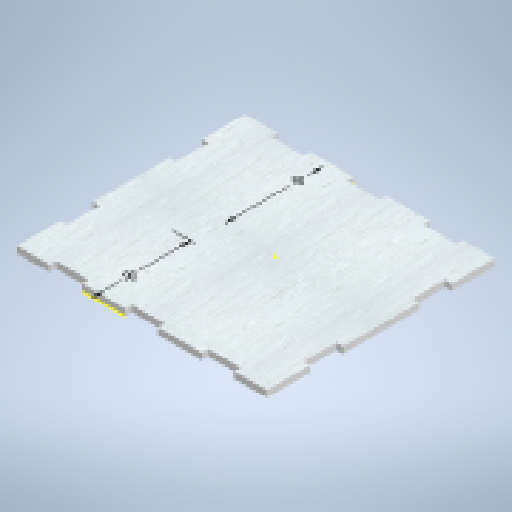
# Autodesk Inventor part: Низ робота
Saved by Autodesk Inventor 2024.2 (Build 282272000, 272)
## iProperties
Created: 2026-01-27
Part Number: Низ робота
Material: Типовые
Document SubType Name: Modeling
Designer: Service
Density: 1 g/cm^3
Appearance: По умолчанию
Author: Service
Autodesk Inventor part; units mm, degrees
ref_plane "YZ Plane" through (0, 0, 0) normal (1, 0, 0) x (0, 1, 0)
ref_plane "XZ Plane" through (0, 0, 0) normal (0, 1, 0) x (-1, 0, 0)
ref_plane "XY Plane" through (0, 0, 0) normal (0, 0, 1) x (1, 0, 0)
sketch "Эскиз1" plane through (0, 0, 0) normal (0, 1, 0) x (-1, 0, 0)
  line L0 (127.5386, 109.5005) -> (-102.4614, 109.5005)
  line L1 (-102.4614, 109.5005) -> (-102.4614, -100.4995)
  line L2 (-102.4614, -100.4995) -> (127.5386, -100.4995)
  line L3 (127.5386, -100.4995) -> (127.5386, 109.5005)
  line L4 (127.5386, -100.4995) -> (97.5386, -100.4995)
  line L5 (97.5386, -100.4995) -> (97.5386, -94.4995)
  line L6 (97.5386, -94.4995) -> (127.5386, -94.4995)
  line L7 (127.5386, -94.4995) -> (127.5386, -100.4995)
  line L8 (97.5386, -94.4995) -> (67.5386, -94.4995)
  line L9 (67.5386, -94.4995) -> (67.5386, -100.4995)
  line L10 (67.5386, -100.4995) -> (97.5386, -100.4995)
  line L11 (97.5386, -100.4995) -> (97.5386, -94.4995)
  line L12 (6.9803, -100.4995) -> (67.5386, -100.4995)
  line L13 (67.5386, -100.4995) -> (67.5386, -94.4995)
  line L14 (-42.4614, -94.4995) -> (-42.4614, -100.4995)
  line L15 (-42.4614, -100.4995) -> (-2.4614, -100.4995)
  line L16 (-42.4614, -94.4995) -> (-72.4614, -94.4995)
  line L17 (-72.4614, -94.4995) -> (-72.4614, -100.4995)
  line L18 (-72.4614, -100.4995) -> (-42.4614, -100.4995)
  line L19 (-42.4614, -100.4995) -> (-42.4614, -94.4995)
  line L20 (-72.4614, -94.4995) -> (-102.4614, -94.4995)
  line L21 (-102.4614, -94.4995) -> (-102.4614, -100.4995)
  line L22 (-102.4614, -100.4995) -> (-72.4614, -100.4995)
  line L23 (-72.4614, -100.4995) -> (-72.4614, -94.4995)
  line L24 (-42.4614, -94.4995) -> (-2.4614, -94.4995)
  line L25 (-2.4614, -94.4995) -> (-2.4614, -100.4995)
  line L26 (-2.4614, -100.4995) -> (-42.4614, -100.4995)
  line L27 (-42.4614, -100.4995) -> (-42.4614, -94.4995)
  line L28 (-2.4614, -100.4995) -> (27.5386, -100.4995)
  line L29 (27.5386, -100.4995) -> (27.5386, -94.4995)
  line L30 (27.5386, -94.4995) -> (-2.4614, -94.4995)
  line L31 (-2.4614, -94.4995) -> (-2.4614, -100.4995)
  line L32 (67.5386, -94.4995) -> (27.5386, -94.4995)
  line L33 (27.5386, -94.4995) -> (27.5386, -100.4995)
  line L34 (27.5386, -100.4995) -> (67.5386, -100.4995)
  line L35 (67.5386, -100.4995) -> (67.5386, -94.4995)
  line L36 (-102.4614, 103.5005) -> (127.5386, 103.5005)
  line L37 (127.5386, 103.5005) -> (97.5386, 103.5005)
  line L38 (97.5386, 103.5005) -> (97.5386, 109.5005)
  line L39 (97.5386, 109.5005) -> (127.5386, 109.5005)
  line L40 (127.5386, 109.5005) -> (127.5386, 103.5005)
  line L41 (97.5386, 109.5005) -> (67.5386, 109.5005)
  line L42 (67.5386, 109.5005) -> (67.5386, 103.5005)
  line L43 (67.5386, 103.5005) -> (97.5386, 103.5005)
  line L44 (97.5386, 103.5005) -> (97.5386, 109.5005)
  line L45 (6.9803, 103.5005) -> (67.5386, 103.5005)
  line L46 (67.5386, 103.5005) -> (67.5386, 109.5005)
  line L47 (-42.4614, 109.5005) -> (-42.4614, 103.5005)
  line L48 (-42.4614, 103.5005) -> (-2.4614, 103.5005)
  line L49 (-42.4614, 109.5005) -> (-72.4614, 109.5005)
  line L50 (-72.4614, 109.5005) -> (-72.4614, 103.5005)
  line L51 (-72.4614, 103.5005) -> (-42.4614, 103.5005)
  line L52 (-42.4614, 103.5005) -> (-42.4614, 109.5005)
  line L53 (-72.4614, 109.5005) -> (-102.4614, 109.5005)
  line L54 (-102.4614, 109.5005) -> (-102.4614, 103.5005)
  line L55 (-102.4614, 103.5005) -> (-72.4614, 103.5005)
  line L56 (-72.4614, 103.5005) -> (-72.4614, 109.5005)
  line L57 (-42.4614, 109.5005) -> (-2.4614, 109.5005)
  line L58 (-2.4614, 109.5005) -> (-2.4614, 103.5005)
  line L59 (-2.4614, 103.5005) -> (-42.4614, 103.5005)
  line L60 (-42.4614, 103.5005) -> (-42.4614, 109.5005)
  line L61 (-2.4614, 103.5005) -> (27.5386, 103.5005)
  line L62 (27.5386, 103.5005) -> (27.5386, 109.5005)
  line L63 (27.5386, 109.5005) -> (-2.4614, 109.5005)
  line L64 (-2.4614, 109.5005) -> (-2.4614, 103.5005)
  line L65 (67.5386, 109.5005) -> (27.5386, 109.5005)
  line L66 (27.5386, 109.5005) -> (27.5386, 103.5005)
  line L67 (27.5386, 103.5005) -> (67.5386, 103.5005)
  line L68 (67.5386, 103.5005) -> (67.5386, 109.5005)
  line L69 (-102.4614, 69.5005) -> (-96.4614, 69.5005)
  line L70 (-96.4614, 69.5005) -> (-96.4614, 39.5005)
  line L71 (-96.4614, 39.5005) -> (-102.4614, 39.5005)
  line L72 (-102.4614, 39.5005) -> (-102.4614, 69.5005)
  line L73 (-102.4614, -30.4995) -> (-96.4614, -30.4995)
  line L74 (-96.4614, -30.4995) -> (-96.4614, -60.4995)
  line L75 (-96.4614, -60.4995) -> (-102.4614, -60.4995)
  line L76 (-102.4614, -60.4995) -> (-102.4614, -30.4995)
  line L77 (127.5386, 69.5005) -> (121.5386, 69.5005)
  line L78 (121.5386, 69.5005) -> (121.5386, 39.5005)
  line L79 (121.5386, 39.5005) -> (127.5386, 39.5005)
  line L80 (127.5386, 39.5005) -> (127.5386, 69.5005)
  line L81 (127.5386, -30.4995) -> (121.5386, -30.4995)
  line L82 (121.5386, -30.4995) -> (121.5386, -60.4995)
  line L83 (121.5386, -60.4995) -> (127.5386, -60.4995)
  line L84 (127.5386, -60.4995) -> (127.5386, -30.4995)
  point P0 (0, 0)
  point P1 (-42.4614, -97.4995)
  point P2 (67.5386, -97.4995)
  point P3 (-42.4614, 106.5005)
  point P4 (67.5386, 106.5005)
  point P5 (-99.4614, -60.4995)
  point P6 (-2.4614, -100.4995)
  point P7 (124.5386, 69.5005)
  point P8 (124.5386, -60.4995)
  dimension "d0" = 230
  dimension "d1" = 210
  dimension "d2" = 6
  dimension "d3" = 30
  dimension "d4" = 30
  dimension "d5" = 30
  dimension "d6" = 30
  dimension "d8" = 40
  dimension "d10" = 40
  dimension "d11" = 230
  dimension "d13" = 6
  dimension "d14" = 30
  dimension "d15" = 30
  dimension "d16" = 30
  dimension "d17" = 30
  dimension "d18" = 40
  dimension "d19" = 40
  dimension "d20" = 40
  dimension "d21" = 30
  dimension "d22" = 40
  dimension "d23" = 30
  dimension "d24" = 6
  dimension "d27" = 6
  dimension "d28" = 40
  dimension "d29" = 40
  dimension "d30" = 30
  dimension "d31" = 30
  constraints: 170 end point, 38 parallel, 19 horizontal, 19 perpendicular, 16 point on line, 7 midpoint
  measures "d0" distance of L1.end L2.end
  measures "d1" distance of L0.end L1.end
  measures "d2" distance of L4.end L5.end
  measures "d3" distance of L5.end L6.end
  measures "d4" distance of L16.end L20.end
  measures "d5" distance of L14.start L16.end
  measures "d6" distance of L5.end L8.end
  measures "d8" distance of L8.end L32.end
  measures "d10" distance of L14.start L24.end
  measures "d11" distance of L55.start L40.end
  measures "d13" distance of L38.start L41.start
  measures "d14" distance of L41.start L39.end
  measures "d15" distance of L53.start L53.end
  measures "d16" distance of L57.start L53.start
  measures "d17" distance of L41.start L42.start
  measures "d18" distance of L42.start L66.start
  measures "d19" distance of L57.start L57.end
  measures "d20" distance from line of point (-99.461, -60.5) L2
  measures "d21" distance of L73.end L74.end
  measures "d22" distance between parallel lines of L69 L0
  measures "d23" distance of L69.end L70.end
  measures "d24" distance of L70.end L71.end
  measures "d27" distance of L78.end L79.end
  measures "d28" distance from line of point (124.539, 69.5) L0
  measures "d29" distance from line of point (124.539, -60.5) L2
  measures "d30" distance of L81.end L82.end
  measures "d31" distance of L77.end L78.end
extrude "Выдавливание1" add sketch "Эскиз1" along normal blind 6 contours L3 L36 L38 L0 | L3 L77 L78 L79 L81 L82 L83 L6 L8 L32 L30 L24 L16 L20 L1 L75 L74 L73 L71 L70 L69 L36 | L42 L36 L62 L0 | L58 L36 L47 L0 | L50 L36 L1 L0 | L3 L2 L5 L6 | L9 L2 L29 L32 | L25 L2 L14 L24 | L17 L2 L1 L20
sketch "Эскиз2" plane through (0, 6, 0) normal (0, 1, 0) x (1, 0, 0)
  point P0 (0, 0)
sketch "Эскиз4" plane through (0, 0, 0) normal (0, -1, 0) x (1, 0, 0)
  line L0 (-86.4691, 58.1623) -> (-86.4691, 34.4995) construction
  line L1 (-86.4691, 34.4995) -> (-89.6455, 34.4995) construction
  line L2 (-89.6455, 34.4995) -> (-89.6455, 58.1623) construction
  line L3 (-89.6455, 58.1623) -> (-86.4691, 58.1623) construction
  line L4 (-75.9914, 19.5005) -> (41.7541, 19.5005)
  line L5 (41.7541, 19.5005) -> (41.7541, 47.0288)
  line L6 (41.7541, 47.0288) -> (80.5935, 4.5005)
  line L7 (80.5935, 4.5005) -> (41.7541, -38.0279)
  line L8 (41.7541, -38.0279) -> (41.7541, -10.4995)
  line L9 (41.7541, -10.4995) -> (-75.9914, -10.4995)
  line L10 (-75.9914, -10.4995) -> (-75.9914, 19.5005)
  line L11 (-67.5386, 109.5005) -> (-27.5386, 109.5005) projected
  line L12 (-27.5386, -100.4995) -> (-67.5386, -100.4995) projected
  point P0 (0, 0)
  dimension "d39" = 90
  dimension "d40" = 90
  constraints: 14 end point, 3 equal length, 3 perpendicular, 1 collinear, 1 horizontal, 2 other
  measures "d39" distance between parallel lines of L11 L4
  measures "d40" distance between parallel lines of L12 L9
